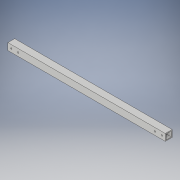
# Autodesk Inventor part: 23in 1x1 Beam
Saved by Autodesk Inventor 2018 (Build 220112000, 112)
## iProperties
Created: 2019-01-16
Part Number: 23in 1x1 Beam
Material: Generic
Document SubType Name: Modeling
Designer: Gabriel
Density: 1 g/cm^3
Appearance: Default
Author: Gabriel
Autodesk Inventor part; units mm, degrees
ref_plane "YZ Plane" through (0, 0, 0) normal (1, 0, 0) x (0, 1, 0)
ref_plane "XZ Plane" through (0, 0, 0) normal (0, 1, 0) x (-1, 0, 0)
ref_plane "XY Plane" through (0, 0, 0) normal (0, 0, 1) x (1, 0, 0)
sketch "Sketch1" plane through (0, 0, 0) normal (1, 0, 0) x (0, 1, 0)
  line L0 (5.4849, 4.7856) -> (-19.9151, 4.7856)
  line L1 (-19.9151, 4.7856) -> (-19.9151, -20.6144)
  line L2 (-19.9151, -20.6144) -> (5.4849, -20.6144)
  line L3 (5.4849, -20.6144) -> (5.4849, 4.7856)
  line L4 (2.3099, 1.6106) -> (-16.7401, 1.6106)
  line L5 (-16.7401, 1.6106) -> (-16.7401, -17.4394)
  line L6 (-16.7401, -17.4394) -> (2.3099, -17.4394)
  line L7 (2.3099, -17.4394) -> (2.3099, 1.6106)
  point P0 (0, 0)
  dimension "d0" = 25.4
  dimension "d1" = 25.4
  dimension "d2" = 3.175
  constraints: 16 end point, 4 parallel, 2 perpendicular, 1 horizontal, 3 other
  measures "d0" distance of L2.end L1.end
  measures "d1" distance of L1.end L0.end
  measures "d2" distance between parallel lines of L3 L7
extrude "Extrusion1" add sketch "Sketch1" along normal blind 584.2
sketch "Sketch3" plane through (0, -19.9151, -20.6144) normal (0, 0, -1) x (-1, 0, 0)
  line L0 (-584.2, 22.225) -> (-584.2, 3.175) construction
  line L1 (-584.2, 12.7) -> (-571.5, 12.7) construction
  line L2 (-571.5, 12.7) -> (-546.1, 12.7) construction
  line L3 (0, 3.175) -> (0, 22.225) construction
  line L4 (0, 12.7) -> (-12.7, 12.7) construction
  line L5 (-12.7, 12.7) -> (-38.1, 12.7) construction
  circle A0 centre (-12.7, 12.7) radius 2.5797
  circle A1 centre (-38.1, 12.7) radius 2.5797
  circle A2 centre (-571.5, 12.7) radius 2.5797
  circle A3 centre (-546.1, 12.7) radius 2.5797
  point P0 (0, 19.9151)
  dimension "d7" = 12.7
  dimension "d8" = 25.4
  dimension "d9" = 12.7
  dimension "d10" = 25.4
  dimension "d11" = 5.1594
  dimension "d12" = 5.1594
  dimension "d13" = 5.1594
  dimension "d14" = 5.1594
  constraints: 8 end point, 4 centre point, 4 coincident, 2 horizontal, 2 midpoint, 2 point on line
  measures "d7" distance of L1.start L1.end
  measures "d8" distance of L1.end L2.end
  measures "d9" distance of L4.start L4.end
  measures "d10" distance of L4.end L5.end
  measures "d11" diameter of A0
  measures "d12" diameter of A1
  measures "d13" diameter of A2
  measures "d14" diameter of A3
extrude "Extrusion3" cut sketch "Sketch3" against normal blind 584.2
body "Solid1"
